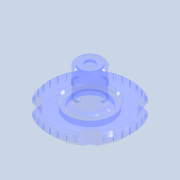
# Autodesk Inventor part: cpd_lowrcf_0.7_p1_v2
Saved by Autodesk Inventor 2021 (Build 250183000, 183)
## iProperties
Created: 2021-12-07
Part Number: cpd_lowrcf_0.7_p1_v2
Material: Generic
Document SubType Name: Modeling
Designer: tomos
Density: 1 g/cm^3
Appearance: Clear - Blue
Author: tomos
Autodesk Inventor part; units mm, degrees
ref_plane "YZ Plane" through (0, 0, 0) normal (1, 0, 0) x (0, 1, 0)
ref_plane "XZ Plane" through (0, 0, 0) normal (0, 1, 0) x (-1, 0, 0)
ref_plane "XY Plane" through (0, 0, 0) normal (0, 0, 1) x (1, 0, 0)
sketch "Sketch1" plane through (0, 0, 0) normal (0, 0, 1) x (1, 0, 0)
  line L0 (0, 0) -> (0, 23.831776) construction
  line L1 (0, 0) -> (13.356698, 0) construction
  line L2 (0, 9.95) -> (1.39, 9.95)
  line L3 (1.39, 9.95) -> (1.39, 9.2)
  line L4 (1.39, 9.2) -> (3, 9.2)
  line L5 (3, 9.2) -> (3, 9.95)
  line L6 (3, 9.95) -> (3.925, 9.95)
  line L7 (3.925, 9.95) -> (3.925, 0)
  line L8 (3.925, 0) -> (12.5, 0)
  line L9 (12.5, 0) -> (12.5, -4)
  line L10 (12.5, -4) -> (0, -4)
  line L11 (0, -4) -> (0, 9.95)
  dimension "d0" = 12.5
  dimension "d1" = 3.925
  dimension "d5" = 3
  dimension "d6" = 0.75
  dimension "d7" = 9.95
  dimension "d8" = 4
  dimension "d35" = 1.39
  constraints: 24 end point, 5 perpendicular, 5 point on line, 2 horizontal, 2 vertical, 1 collinear
  measures "d0" distance between parallel lines of L9 L0
  measures "d1" distance between parallel lines of L7 L0
  measures "d5" distance between parallel lines of L5 L0
  measures "d6" distance between parallel lines of L2 L4
  measures "d7" distance between parallel lines of L1 L6
  measures "d8" distance between parallel lines of L1 L10
  measures "d35" distance between parallel lines of L3 L0
sketch "Sketch1 outline for Revolution1" plane through (0, 0, 0) normal (0, 0, 1) x (1, 0, 0)
  line L0 (0, 9.95) -> (0, -4)
  line L1 (1.39, 9.95) -> (0, 9.95)
  line L2 (1.39, 9.2) -> (1.39, 9.95)
  line L3 (3, 9.2) -> (1.39, 9.2)
  line L4 (3, 9.95) -> (3, 9.2)
  line L5 (3.925, 9.95) -> (3, 9.95)
  line L6 (3.925, 0) -> (3.925, 9.95)
  line L7 (12.5, 0) -> (3.925, 0)
  line L8 (12.5, -4) -> (12.5, 0)
  line L9 (0, -4) -> (12.5, -4)
revolve "Revolution1" add sketch "Sketch1 outline for Revolution1" angle 360 about axis through (0, 0, 0) along (0, 1, 0)
chamfer "Chamfer1" distance 2 angle 45 1 edges at (-12.5, -4, 0)
chamfer "Chamfer2" distance 1 angle 45 1 edges at (-12.5, 0, 0)
sketch "Sketch4" plane through (0, 0, 0) normal (0, 1, 0) x (1, 0, 0)
  circle A0 centre (0, 0) radius 3.925
  line L0 (0, 0) -> (0, -6.745083) construction
  line L1 (-1, -3.795474) -> (-1, -4.822409)
  circle A1 centre (0, 0) radius 4.925
  line L2 (1, -3.795474) -> (1, -4.822409)
  circle A2 centre (0, 0) radius 3.925
  point P0 (1, -6.119865)
  dimension "d19" = 7.85
  dimension "d20" = 9.85
  dimension "d21" = 1
  constraints: 6 end point, 4 coincident, 2 centre point, 2 point on circle, 2 symmetric about line, 2 vertical, 2 other
  measures "d19" diameter of A0
  measures "d20" diameter of A1
  measures "d21" distance between parallel lines of L1 L0
sketch "Sketch4 outline for Extrusion1" plane through (0, 0, 0) normal (0, 1, 0) x (1, 0, 0)
  line L0 (1, -4.822409) -> (1, -3.795474)
  arc A0 (-1, -4.822409) -> (1, -4.822409) centre (0, 0) ccw
  line L1 (-1, -3.795474) -> (-1, -4.822409)
  arc A1 (1, -3.795474) -> (-1, -3.795474) centre (0, 0) cw
extrude "Extrusion1" add sketch "Sketch4 outline for Extrusion1" along normal blind 4
sketch "Sketch5" plane through (0, 0, 0) normal (1, 0, 0) x (0, 1, 0)
  line L0 (0, 0) -> (0, 9.63585) construction
  line L1 (0, 0) -> (7.566624, 0) construction
  line L2 (0, 3.925) -> (4.45214, 3.925) construction
  line L3 (0, 3.925) -> (2.25, 3.925)
  line L4 (2.25, 3.925) -> (2.25, 5.925)
  line L5 (2.25, 5.925) -> (0, 5.925)
  line L6 (0, 5.925) -> (0, 3.925)
  dimension "d24" = 3.925
  dimension "d25" = 2.25
  dimension "d26" = 2
  constraints: 14 end point, 3 horizontal, 2 parallel, 1 perpendicular, 1 point on line, 1 vertical
  measures "d24" distance between parallel lines of L1 L2
  measures "d25" distance between parallel lines of L4 L0
  measures "d26" distance between parallel lines of L2 L5
sketch "Sketch5 outline for Revolution2" plane through (0, 0, 0) normal (1, 0, 0) x (0, 1, 0)
  line L0 (0, 3.925) -> (2.25, 3.925)
  line L1 (0, 5.925) -> (0, 3.925)
  line L2 (2.25, 5.925) -> (0, 5.925)
  line L3 (2.25, 3.925) -> (2.25, 5.925)
revolve "Revolution2" cut sketch "Sketch5 outline for Revolution2" angle 360 about axis through (0, 0, 0) along (0, 1, 0)
pattern_circular "Circular Pattern1" count 4 over 360 about axis through (0, -10, 0) along (0, 1, 0) of "Extrusion1", "Revolution2"
fillet "Fillet1" radius 0.25 8 edges at (1, 4, 4.3089) (-1, 4, 4.3089) (-1, 2.25, 4.3089) (0, 4, 4.925) (-1, 3.125, 4.8224) (0, 2.25, 4.925) (1, 2.25, 4.3089) (1, 3.125, 4.8224)
pattern_circular "Circular Pattern2" count 4 over 360 about axis through (0, -10, 0) along (0, 1, 0) of "Fillet1"
chamfer "Chamfer3" distance 0.5 angle 45 1 edges at (-3.925, 9.95, 0)
sketch "Sketch6" plane through (0, -4, 0) normal (0, -1, 0) x (1, 0, 0)
  circle A0 centre (0, 0) radius 12.5
  circle A1 centre (0, 0) radius 12
  line L0 (0, 0) -> (-3.64138, 0) construction
  line L1 (-11.997396, 0.25) -> (-12.4975, 0.25)
  line L2 (-11.997396, -0.25) -> (-12.4975, -0.25)
  point P0 (-12.4975, -0.25)
  dimension "d40" = 25
  dimension "d41" = 24
  dimension "d39" = 0.25
  constraints: 6 end point, 3 coincident, 2 horizontal, 2 symmetric about line, 6 other
  measures "d39" distance between parallel lines of L1 L0
sketch "Sketch6 outline for Extrusion2" plane through (0, -4, 0) normal (0, -1, 0) x (1, 0, 0)
  line L0 (-12.4975, -0.25) -> (-11.997396, -0.25)
  arc A0 (-12.4975, 0.25) -> (-12.4975, -0.25) centre (0, 0) ccw
  line L1 (-11.997396, 0.25) -> (-12.4975, 0.25)
  arc A1 (-11.997396, -0.25) -> (-11.997396, 0.25) centre (0, 0) cw
extrude "Extrusion2" cut sketch "Sketch6 outline for Extrusion2" against normal through all
pattern_circular "Circular Pattern3" count 36 over 360 about axis through (0, -10, 0) along (0, 1, 0) of "Extrusion2"
sketch "Sketch7" plane through (0, 0, 0) normal (0, 0, 1) x (1, 0, 0)
  line L0 (0, 0) -> (7.517894, 0) construction
  line L1 (0, 0) -> (0, 6.549744) construction
  line L2 (6.575, 0) -> (5.175, 0)
  line L3 (5.175, 0) -> (5.175, -2)
  line L4 (5.175, -2) -> (6.575, -2)
  line L5 (6.575, -2) -> (6.575, 0)
  dimension "d47" = 6.575
  dimension "d48" = 5.175
  dimension "d49" = 2
  constraints: 12 end point, 2 horizontal, 2 parallel, 1 perpendicular, 1 point on line, 1 vertical
  measures "d47" distance between parallel lines of L1 L5
  measures "d48" distance between parallel lines of L1 L3
  measures "d49" distance between parallel lines of L4 L0
sketch "Sketch7 outline for Revolution3" plane through (0, 0, 0) normal (0, 0, 1) x (1, 0, 0)
  line L0 (6.575, 0) -> (5.175, 0)
  line L1 (6.575, -2) -> (6.575, 0)
  line L2 (5.175, -2) -> (6.575, -2)
  line L3 (5.175, 0) -> (5.175, -2)
revolve "Revolution3" cut sketch "Sketch7 outline for Revolution3" angle 360 about axis through (0, 0, 0) along (0, 1, 0)
sketch "Sketch8" plane through (0, 0, 0) normal (0, 1, 0) x (1, 0, 0)
  circle A0 centre (0, 0) radius 12.5
  circle A1 centre (0, 0) radius 1.39 construction
  line L0 (0, 0) -> (0, 16.625394) construction
  line L1 (0, 0) -> (13.524085, 13.524085) construction
  circle A2 centre (8.838835, 8.838835) radius 2.5
  point P0 (6.903152, 10.420964)
  point P1 (10.420964, 6.903152)
  dimension "d54" = 25
  dimension "d58" = 45
  dimension "d59" = 5
  constraints: 4 end point, 1 centre point, 1 coincident, 1 point on line, 1 vertical, 3 other
  measures "d58" angle of L1 L0
  measures "d59" diameter of A2
sketch "Sketch8 outline for Extrusion3" plane through (0, 0, 0) normal (0, 1, 0) x (1, 0, 0)
  arc A0 (6.903152, 10.420964) -> (10.420964, 6.903152) centre (8.838835, 8.838835) ccw
  arc A1 (10.420964, 6.903152) -> (6.903152, 10.420964) centre (0, 0) ccw
extrude "Extrusion3" cut sketch "Sketch8 outline for Extrusion3" against normal through all
chamfer "Chamfer4" distance 0.5 angle 45 2 edges at (-6.575, 0, 0) (-5.175, 0, 0)
pattern_circular "Circular Pattern4" count 4 over 360 about axis through (0, -10, 0) along (0, 1, 0) of "Extrusion3"
body "Solid1"
